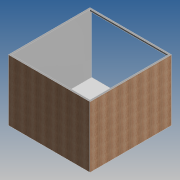
# Autodesk Inventor part: P001_CageDeTest
Saved by Autodesk Inventor 2020 (Build 240168000, 168)
## iProperties
Created: 2021-09-24
Part Number: P001_CageDeTest
Material: Générique
Document SubType Name: Modeling
Designer: gabri
Density: 1 g/cm^3
Appearance: Par défaut
Author: gabri
Autodesk Inventor part; units mm, degrees
ref_plane "YZ Plane" through (0, 0, 0) normal (1, 0, 0) x (0, 1, 0)
ref_plane "XZ Plane" through (0, 0, 0) normal (0, 1, 0) x (-1, 0, 0)
ref_plane "XY Plane" through (0, 0, 0) normal (0, 0, 1) x (1, 0, 0)
sketch "Esquisse2" plane through (0, 0, 0) normal (0, 0, 1) x (1, 0, 0)
  line L0 (-1000, 1000) -> (1000, 1000)
  line L1 (1000, 1000) -> (1000, -1000)
  line L2 (1000, -1000) -> (-1000, -1000)
  line L3 (-1000, -1000) -> (-1000, 1000)
  line L4 (0, 1400) -> (0, -1400) construction
  line L5 (-1400, 0) -> (1400, 0) construction
  point P0 (0, 0)
  dimension "d0" = 2000
  dimension "d1" = 2000
  dimension "d2" = 1000
  dimension "d3" = 1000
  constraints: 8 end point, 2 parallel, 1 horizontal, 1 perpendicular
  measures "d0" distance of L2.end L0.start
  measures "d1" distance of L1.end L2.end
  measures "d2" distance between parallel lines of L4 L1
  measures "d3" distance between parallel lines of L5 L0
extrude "Extrusion1" add sketch "Esquisse2" along normal blind 1500
sketch "Esquisse3" plane through (-1000, 1000, 0) normal (0, 1, 0) x (1, 0, 0)
  line L0 (2000, 0) -> (0, 0) construction
  line L1 (0, 0) -> (0, -1500) construction
  line L2 (2000, -1500) -> (0, -1500) construction
  line L3 (2000, 0) -> (2000, -1500) construction
  line L4 (40, -1460) -> (1960, -1460)
  line L5 (1960, -1460) -> (1960, -40)
  line L6 (1960, -40) -> (40, -40)
  line L7 (40, -40) -> (40, -1460)
  point P0 (1000, 0)
  dimension "d6" = 1920
  dimension "d8" = 40
  dimension "d9" = 40
  dimension "d21" = 40
  constraints: 8 end point, 2 parallel, 1 horizontal, 1 perpendicular
  measures "d6" distance of L4.start L4.end
  measures "d8" distance between parallel lines of L1 L7
  measures "d9" distance between parallel lines of L2 L4
  measures "d21" distance between parallel lines of L0 L6
extrude "Extrusion2" cut sketch "Esquisse3" against normal blind 1960
sketch "Esquisse5" plane through (960, 1000, 1460) normal (0, 0, -1) x (-1, 0, 0)
  line L0 (0, 0) -> (1920, 0) construction
  line L1 (0, 0) -> (0, -1960) construction
  line L2 (0, -1960) -> (1920, -1960) construction
  line L3 (1920, 0) -> (1920, -1960) construction
  line L4 (0, -1960) -> (1920, -1960) construction
  line L5 (1920, 0) -> (0, 0)
  line L6 (0, 0) -> (0, -1960)
  line L7 (0, -1960) -> (1920, -1960)
  line L8 (1920, -1960) -> (1920, 0)
  point P0 (960, -1000)
  constraints: 8 end point, 2 parallel, 1 horizontal, 1 perpendicular
extrude "Extrusion4" cut sketch "Esquisse5" against normal blind 40
sketch "Esquisse6" plane through (1000, -1000, 0) normal (1, 0, 0) x (0, 0, -1)
  line L0 (0, 0) -> (0, 2000) construction
  line L1 (0, 2000) -> (-1500, 2000) construction
  line L2 (-1500, 0) -> (-1500, 2000) construction
  line L3 (0, 0) -> (-1500, 0) construction
  line L4 (-1500, 2000) -> (-1460, 2000)
  line L5 (-1460, 2000) -> (-1460, 1960)
  line L6 (-1460, 1960) -> (-1500, 1960)
  line L7 (-1500, 1960) -> (-1500, 2000)
  point P0 (0, 1000)
  dimension "d16" = 40
  dimension "d17" = 40
  constraints: 8 end point, 2 parallel, 1 horizontal, 1 perpendicular
  measures "d16" distance of L5.end L6.end
  measures "d17" distance between parallel lines of L1 L6
extrude "Extrusion5" add sketch "Esquisse6" against normal blind 2000
